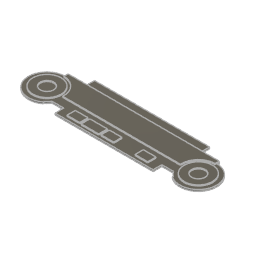
Face test plate (Autodesk Fusion 360 design; units mm, degrees)
Autodesk Fusion 360 part; units mm, degrees
sketch "Sketch1" plane through (0, 0, 0) normal (0, 0, 1) x (1, 0, 0)
  line L0 (110.9582, 1.828) -> (110.9582, -11.672)
  line L1 (-73.5418, 1.828) -> (-73.5418, -11.672)
  line L2 (-73.5418, -24.672) -> (110.9582, -24.672)
  line L3 (-73.5418, 15.328) -> (110.9582, 15.328)
  line L4 (110.9582, -24.672) -> (130.9582, -24.672)
  line L5 (130.9582, -24.672) -> (130.9582, -11.672)
  line L6 (130.9582, 15.328) -> (110.9582, 15.328)
  line L7 (-73.5418, 15.328) -> (-93.5418, 15.328)
  line L8 (-93.5418, -4.672) -> (-93.5418, -24.672)
  line L9 (-93.5418, -24.672) -> (-73.5418, -24.672)
  line L10 (130.9582, -4.672) -> (150.3831, -4.672)
  line L11 (130.9582, 15.328) -> (150.3831, 15.328)
  line L12 (-93.5418, -24.672) -> (-93.5418, -24)
  line L13 (-93.5418, -4.672) -> (-112.9667, -4.672)
  line L14 (-93.5418, 15.328) -> (-112.9667, 15.328)
  line L15 (130.9582, -4.672) -> (130.9582, -11.672)
  line L16 (-112.9667, 85.328) -> (-110, 85.328)
  line L17 (-110, 85.328) -> (150.3831, 85.328)
  line L18 (18.7082, 66.328) -> (150.3831, 66.328)
  line L19 (18.7082, 66.328) -> (16.2618, 66.328)
  line L20 (16.2618, 66.328) -> (-112.9667, 66.328)
  line L21 (157.4958, -4.672) -> (150.3831, -4.672)
  line L22 (191.7412, -4.672) -> (190, -4.672)
  line L23 (-112.9667, -4.672) -> (-120.0796, -4.672)
  circle A0 centre (191.7412, 17.8726) radius 32.5
  circle A1 centre (-154.3247, 17.873) radius 32.5
  line L24 (-112.9667, 66.328) -> (-154.3247, 66.328)
  line L25 (-154.3247, 66.328) -> (-154.3247, 60.373)
  line L26 (150.3831, 66.328) -> (191.7412, 66.328)
  line L27 (191.7412, 66.328) -> (191.7412, 60.3726)
  line L28 (150.3831, 66.328) -> (150.3831, 85.328)
  line L29 (150.3831, 15.328) -> (153.3253, 15.328)
  line L30 (191.7412, 60.3726) -> (191.7412, 56.3726)
  arc A2 (157.4958, -4.672) -> (166.8041, -14.672) centre (191.7412, 17.8726) ccw
  arc A3 (191.7412, 56.3726) -> (153.3253, 15.328) centre (191.7412, 17.8726) ccw
  line L31 (-112.9667, 66.328) -> (-112.9667, 85.328)
  line L32 (-154.3247, 60.373) -> (-154.3247, 56.373)
  line L33 (-112.9667, 15.328) -> (-115.9089, 15.328)
  arc A4 (-154.3247, 60.373) -> (-128.382, -15.7904) centre (-154.3247, 17.873) ccw
  arc A5 (-129.3883, -14.672) -> (-120.0796, -4.672) centre (-154.3247, 17.873) ccw
  arc A6 (-115.9089, 15.328) -> (-154.3247, 56.373) centre (-154.3247, 17.873) ccw
  line L34 (130.9582, -24.672) -> (130.9582, -14.672)
  line L35 (165.7979, -15.7904) -> (166.8041, -14.672)
  line L36 (-129.3883, -14.672) -> (-128.382, -15.7904)
  arc A7 (165.7979, -15.7904) -> (233.946, 12.8726) centre (191.7412, 17.8726) ccw
  arc A8 (233.946, 22.8726) -> (191.7412, 60.3726) centre (191.7412, 17.8726) ccw
  line L37 (110.9582, 1.828) -> (81.9582, 1.828)
  line L38 (81.9582, 1.828) -> (81.9582, -17.172)
  line L39 (81.9582, -17.172) -> (110.9582, -17.172)
  line L40 (110.9582, -17.172) -> (110.9582, -11.672)
  line L41 (-73.5418, 1.828) -> (-44.5418, 1.828)
  line L42 (-44.5418, 1.828) -> (-44.5418, -17.172)
  line L43 (-44.5418, -17.172) -> (-73.5418, -17.172)
  line L44 (-73.5418, -17.172) -> (-73.5418, -11.672)
  line L45 (33.2082, 1.828) -> (4.2082, 1.828)
  line L46 (33.2082, 1.828) -> (33.2082, -17.172)
  line L47 (33.2082, -17.172) -> (4.2082, -17.172)
  line L48 (4.2082, -17.172) -> (4.2082, 1.828)
  line L49 (-0.1668, 1.828) -> (-40.1668, 1.828)
  line L50 (-0.1668, 1.828) -> (-0.1668, -18.172)
  line L51 (-0.1668, -18.172) -> (-40.1668, -18.172)
  line L52 (-40.1668, -18.172) -> (-40.1668, 1.828)
  line L53 (233.946, 22.8726) -> (233.946, 12.8726)
  circle A9 centre (-154.3247, 17.873) radius 15.5
  circle A10 centre (191.7412, 17.8726) radius 15.5
  dimension "d9" = 13
  dimension "d10" = 13
  dimension "d12" = 13.5
  dimension "d13" = 13.5
  dimension "d14" = 20
  dimension "d15" = 20
  dimension "d16" = 20
  dimension "d17" = 20
  dimension "d50" = 70
  dimension "d51" = 70
  dimension "d57" = 65
  dimension "d58" = 77
  dimension "d59" = 65
  dimension "d60" = 77
  dimension "d61" = 82
  dimension "d63" = 82
  dimension "d64" = 85
  dimension "d65" = 10
  dimension "d68" = 29
  dimension "d69" = 19
  dimension "d70" = 29
  dimension "d71" = 19
  dimension "d73" = 29
  dimension "d74" = 19
  dimension "d76" = 40
  dimension "d77" = 20
  dimension "d78" = 40
  dimension "d79" = 31
  dimension "d80" = 31
  constraint vertical L0
  constraint vertical L1
  constraint perpendicular L2 L8
  constraint coincident L8 L12.end
  constraint perpendicular L9 L12
  constraint perpendicular L8 L13
  constraint perpendicular L8 L14
  constraint perpendicular L10 L15
  constraint perpendicular L16 L31
  constraint perpendicular L17 L28
  constraint perpendicular L18 L28
  constraint perpendicular L20 L31
  constraint coincident L21 L22.end
  constraint concentric A0 A3
  constraint concentric A1 A6
  constraint concentric A2 A3
  constraint concentric A1 A5
  constraint concentric A1 A4
  constraint horizontal L24
  constraint perpendicular L24 L25
  constraint perpendicular L25 L26
  constraint perpendicular L26 L27
  constraint vertical L30
  constraint vertical L32
  constraint perpendicular L4 L34
  constraint concentric A7 A8
  constraint perpendicular L0 L37
  constraint perpendicular L0 L39
  constraint perpendicular L1 L43
  constraint perpendicular L43 L44
  constraint perpendicular L46 L47
  constraint perpendicular L49 L50
  constraint perpendicular L50 L51
  constraint concentric A4 A9
  constraint concentric A2 A10
  measures "d9" distance of L0.end L2.end
  measures "d10" distance of L1.end L2.start
  measures "d12" distance of L0.start L3.end
  measures "d13" distance of L1.start L3.start
  measures "d14" distance of L0.end L5.end
  measures "d15" distance of L2.end L4.end
  measures "d16" distance of L3.start L7.end
  measures "d17" distance of L6.start L10.start
  measures "d50" distance of L11.end L17.end
  measures "d51" distance of L14.end L16.start
  measures "d57" diameter of A0
  measures "d58" diameter of A3
  measures "d59" diameter of A1
  measures "d60" diameter of A6
  measures "d61" diameter of A2
  measures "d63" diameter of A5
  measures "d64" diameter of A4
  measures "d65" distance of L4.end L34.end
  measures "d68" distance of L0.start L37.end
  measures "d69" distance of L37.end L38.end
  measures "d70" distance of L1.start L41.end
  measures "d71" distance of L41.end L42.end
  measures "d73" distance of L45.start L45.end
  measures "d74" distance of L45.start L46.end
  measures "d76" distance of L49.start L49.end
  measures "d77" distance of L49.start L50.end
  measures "d78" distance of L50.end L51.end
  measures "d79" diameter of A9
  measures "d80" diameter of A10
extrude "Extrude1" add sketch "Sketch1" along normal blind 4 contours L0 L37 L38 L39 L40 | L1 L41 L42 L43 L44 | L2 L3 L4 L5 L6 L7 L8 L9 L10 L11 L12 L13 L14 L15 L21 L23 L29 L30 A2 A3 L32 L33 A4 A5 A6 L34 L35 L36 A7 A8 L53 | L3 L6 L7 L11 L14 L18 L19 L20 L24 L25 L26 L27 L29 L30 A3 L32 L33 A6 | L16 L17 L18 L19 L20 L28 L31 | A0 | A1 | L45 L46 L47 L48 | L49 L50 L51 L52 | A9 | A10
sketch "Sketch2" plane through (0, 0, 4) normal (0, 0, 1) x (-1, 0, 0)
  line L0 (-150.3831, -66.328) -> (-150.3831, -85.328)
  line L1 (-150.3831, -85.328) -> (112.9667, -85.328)
  line L2 (112.9667, -85.328) -> (112.9667, -66.328)
  line L3 (112.9667, -66.328) -> (154.3247, -66.328)
  line L4 (154.3247, -66.328) -> (154.3247, -60.373)
  arc A0 (154.3247, -60.373) -> (128.382, 15.7904) centre (154.3247, -17.873) ccw
  line L5 (128.382, 15.7904) -> (129.3883, 14.672)
  arc A1 (129.3883, 14.672) -> (120.0796, 4.672) centre (154.3247, -17.873) ccw
  line L6 (120.0796, 4.672) -> (93.5418, 4.672)
  line L7 (93.5418, 4.672) -> (93.5418, 24.672)
  line L8 (93.5418, 24.672) -> (-130.9582, 24.672)
  line L9 (-130.9582, 24.672) -> (-130.9582, 4.672)
  line L10 (-130.9582, 4.672) -> (-157.4958, 4.672)
  arc A2 (-157.4958, 4.672) -> (-166.8041, 14.672) centre (-191.7412, -17.8726) ccw
  line L11 (-166.8041, 14.672) -> (-165.7979, 15.7904)
  arc A3 (-165.7979, 15.7904) -> (-233.946, -12.8726) centre (-191.7412, -17.8726) ccw
  line L12 (-233.946, -12.8726) -> (-233.946, -22.8726)
  arc A4 (-233.946, -22.8726) -> (-191.7412, -60.3726) centre (-191.7412, -17.8726) ccw
  line L13 (-191.7412, -60.3726) -> (-191.7412, -66.328)
  line L14 (-191.7412, -66.328) -> (-150.3831, -66.328)
  arc A5 (-191.6728, -56.4374) -> (-153.2569, -15.3929) centre (-191.6728, -17.9374) ccw
  line L15 (154.393, -66.3929) -> (154.393, -60.4379)
  line L16 (73.6102, -15.3929) -> (-110.8898, -15.3929)
  line L17 (113.035, -66.3929) -> (113.035, -85.3929)
  line L18 (40.2352, 18.1071) -> (40.2352, -1.8929)
  line L19 (110.0684, -85.3929) -> (-150.3147, -85.3929)
  line L20 (0.2352, 18.1071) -> (40.2352, 18.1071)
  line L21 (-33.1398, -1.8929) -> (-33.1398, 17.1071)
  line L22 (-16.1934, -66.3929) -> (113.035, -66.3929)
  arc A6 (154.393, -60.4379) -> (128.4504, 15.7255) centre (154.393, -17.9379) ccw
  line L23 (-18.6398, -66.3929) -> (-150.3147, -66.3929)
  line L24 (73.6102, 24.6071) -> (-110.8898, 24.6071)
  arc A7 (129.4567, 14.6071) -> (120.148, 4.6071) centre (154.393, -17.9379) ccw
  line L25 (113.035, -66.3929) -> (154.393, -66.3929)
  line L26 (73.6102, -15.3929) -> (93.6102, -15.3929)
  line L27 (113.035, -15.3929) -> (115.9772, -15.3929)
  line L28 (113.035, 4.6071) -> (120.148, 4.6071)
  line L29 (93.6102, 4.6071) -> (113.035, 4.6071)
  line L30 (93.6102, 24.6071) -> (93.6102, 23.9351)
  line L31 (44.6102, 17.1071) -> (73.6102, 17.1071)
  line L32 (93.6102, 4.6071) -> (93.6102, 24.6071)
  line L33 (0.2352, -1.8929) -> (0.2352, 18.1071)
  line L34 (73.6102, -1.8929) -> (44.6102, -1.8929)
  line L35 (93.6102, 24.6071) -> (73.6102, 24.6071)
  line L36 (73.6102, 17.1071) -> (73.6102, 11.6071)
  line L37 (-18.6398, -66.3929) -> (-16.1934, -66.3929)
  line L38 (129.4567, 14.6071) -> (128.4504, 15.7255)
  line L39 (73.6102, -1.8929) -> (73.6102, 11.6071)
  line L40 (154.393, -60.4379) -> (154.393, -56.4379)
  line L41 (-4.1398, 17.1071) -> (-4.1398, -1.8929)
  line L42 (44.6102, -1.8929) -> (44.6102, 17.1071)
  line L43 (113.035, -85.3929) -> (110.0684, -85.3929)
  line L44 (93.6102, -15.3929) -> (113.035, -15.3929)
  line L45 (-33.1398, 17.1071) -> (-4.1398, 17.1071)
  line L46 (-33.1398, -1.8929) -> (-4.1398, -1.8929)
  line L47 (0.2352, -1.8929) -> (40.2352, -1.8929)
  circle A8 centre (-191.6728, -17.9374) radius 15.5
  line L48 (-110.8898, -1.8929) -> (-81.8898, -1.8929)
  line L49 (-191.6728, -60.4374) -> (-191.6728, -56.4374)
  line L50 (-130.8898, 4.6071) -> (-150.3147, 4.6071)
  line L51 (-130.8898, -15.3929) -> (-110.8898, -15.3929)
  line L52 (-81.8898, -1.8929) -> (-81.8898, 17.1071)
  arc A9 (-233.8776, -22.9374) -> (-191.6728, -60.4374) centre (-191.6728, -17.9374) ccw
  circle A10 centre (-191.6728, -17.9374) radius 32.5
  line L53 (-130.8898, 24.6071) -> (-130.8898, 11.6071)
  arc A11 (-157.4274, 4.6071) -> (-166.7357, 14.6071) centre (-191.6728, -17.9374) ccw
  line L54 (-157.4274, 4.6071) -> (-150.3147, 4.6071)
  line L55 (-110.8898, 24.6071) -> (-130.8898, 24.6071)
  line L56 (-130.8898, -15.3929) -> (-150.3147, -15.3929)
  line L57 (-110.8898, 17.1071) -> (-110.8898, 11.6071)
  line L58 (-165.7295, 15.7255) -> (-166.7357, 14.6071)
  line L59 (-191.6728, -66.3929) -> (-191.6728, -60.4374)
  line L60 (-130.8898, 24.6071) -> (-130.8898, 14.6071)
  line L61 (-81.8898, 17.1071) -> (-110.8898, 17.1071)
  arc A12 (-165.7295, 15.7255) -> (-233.8776, -12.9374) centre (-191.6728, -17.9374) ccw
  line L62 (-150.3147, -15.3929) -> (-153.2569, -15.3929)
  line L63 (-233.8776, -22.9374) -> (-233.8776, -12.9374)
  line L64 (-110.8898, -1.8929) -> (-110.8898, 11.6071)
  line L65 (-150.3147, -66.3929) -> (-150.3147, -85.3929)
  line L66 (-130.8898, 4.6071) -> (-130.8898, 11.6071)
  line L67 (-150.3147, -66.3929) -> (-191.6728, -66.3929)
  circle A13 centre (154.393, -17.9379) radius 32.5
  circle A14 centre (154.393, -17.9379) radius 15.5
  arc A15 (115.9772, -15.3929) -> (154.393, -56.4379) centre (154.393, -17.9379) ccw
  point P0 (0.0684, -0.0649)
  dimension "d83" = 13
  dimension "d84" = 13
  dimension "d85" = 13.5
  dimension "d86" = 13.5
  dimension "d87" = 20
  dimension "d88" = 20
  dimension "d89" = 20
  dimension "d90" = 20
  dimension "d91" = 70
  dimension "d92" = 70
  dimension "d93" = 65
  dimension "d94" = 77
  dimension "d95" = 65
  dimension "d96" = 77
  dimension "d97" = 82
  dimension "d98" = 82
  dimension "d99" = 85
  dimension "d100" = 10
  dimension "d101" = 29
  dimension "d102" = 19
  dimension "d103" = 29
  dimension "d104" = 19
  dimension "d105" = 29
  dimension "d106" = 19
  dimension "d107" = 40
  dimension "d108" = 20
  dimension "d109" = 40
  dimension "d110" = 31
  dimension "d111" = 31
  constraint perpendicular L24 L32
  constraint coincident L30.end L32
  constraint perpendicular L30 L35
  constraint perpendicular L29 L32
  constraint perpendicular L32 L44
  constraint perpendicular L50 L66
  constraint perpendicular L17 L43
  constraint perpendicular L19 L65
  constraint perpendicular L23 L65
  constraint perpendicular L17 L22
  constraint concentric A5 A10
  constraint concentric A13 A15
  constraint concentric A5 A11
  constraint concentric A7 A13
  constraint concentric A6 A13
  constraint perpendicular L15 L25
  constraint perpendicular L15 L67
  constraint perpendicular L59 L67
  constraint perpendicular L55 L60
  constraint concentric A9 A12
  constraint perpendicular L48 L64
  constraint perpendicular L61 L64
  constraint perpendicular L31 L39
  constraint perpendicular L31 L36
  constraint perpendicular L21 L45
  constraint perpendicular L33 L47
  constraint perpendicular L20 L33
  constraint concentric A6 A14
  constraint concentric A8 A11
  measures "d83" distance of L24.end L57.end
  measures "d84" distance of L36.end L24.start
  measures "d85" distance of L48.start L16.end
  measures "d86" distance of L34.start L16.start
  measures "d87" distance of L57.end L53.end
  measures "d88" distance of L24.end L53.start
  measures "d89" distance of L16.start L26.end
  measures "d90" distance of L51.start L50.start
  measures "d91" distance of L19.end L56.end
  measures "d92" distance of L27.start L17.end
  measures "d93" diameter of A10
  measures "d94" diameter of A5
  measures "d95" diameter of A13
  measures "d96" diameter of A15
  measures "d97" diameter of A11
  measures "d98" diameter of A7
  measures "d99" diameter of A6
  measures "d100" distance of L53.start L60.end
  measures "d101" distance of L48.start L48.end
  measures "d102" distance of L48.end L52.end
  measures "d103" distance of L34.start L34.end
  measures "d104" distance of L34.end L31.start
  measures "d105" distance of L41.end L21.start
  measures "d106" distance of L21.end L21.start
  measures "d107" distance of L18.end L33.start
  measures "d108" distance of L20.start L33.start
  measures "d109" distance of L20.start L18.start
  measures "d110" diameter of A14
  measures "d111" diameter of A8
extrude "Extrude2" add sketch "Sketch2" along normal blind 2 contours L0 L2 L3 L4 A0 L14 A5 L16 L22 L23 L26 L27 L37 L40 L44 L49 L51 L56 L59 L62 L67 A15
sketch "Sketch3" plane through (0, 0, 4) normal (0, 0, 1) x (-1, 0, 0)
  line L0 (-191.6728, -66.328) -> (-191.6728, -56.4374)
  arc A0 (-191.6728, -56.4374) -> (-153.2569, -15.3929) centre (-191.6728, -17.9374) ccw
  line L1 (-153.2569, -15.3929) -> (115.9772, -15.3929)
  arc A1 (115.9772, -15.3929) -> (154.393, -56.4379) centre (154.393, -17.9379) ccw
  line L2 (154.393, -56.4379) -> (154.393, -60.373)
  arc A2 (154.393, -60.373) -> (128.382, 15.7904) centre (154.3247, -17.873) ccw
  line L3 (128.382, 15.7904) -> (129.3883, 14.672)
  arc A3 (129.3883, 14.672) -> (120.0796, 4.672) centre (154.3247, -17.873) ccw
  line L4 (120.0796, 4.672) -> (93.5418, 4.672)
  line L5 (93.5418, 4.672) -> (93.5418, 24.672)
  line L6 (93.5418, 24.672) -> (-130.9582, 24.672)
  line L7 (-130.9582, 24.672) -> (-130.9582, 4.672)
  line L8 (-130.9582, 4.672) -> (-157.4958, 4.672)
  arc A4 (-157.4958, 4.672) -> (-166.8041, 14.672) centre (-191.7412, -17.8726) ccw
  line L9 (-166.8041, 14.672) -> (-165.7979, 15.7904)
  arc A5 (-165.7979, 15.7904) -> (-233.946, -12.8726) centre (-191.7412, -17.8726) ccw
  line L10 (-233.946, -12.8726) -> (-233.946, -22.8726)
  arc A6 (-233.946, -22.8726) -> (-191.7412, -60.3726) centre (-191.7412, -17.8726) ccw
  line L11 (-191.7412, -60.3726) -> (-191.7412, -66.328)
  line L12 (-191.7412, -66.328) -> (-191.6728, -66.328)
  arc A7 (-191.7975, -56.4377) -> (-153.3817, -15.3932) centre (-191.7975, -17.9377) ccw
  line L13 (154.2683, -66.3932) -> (154.2683, -60.4382)
  line L14 (73.4855, -15.3932) -> (-111.0145, -15.3932)
  line L15 (112.9103, -66.3932) -> (112.9103, -85.3932)
  line L16 (40.1105, 18.1068) -> (40.1105, -1.8932)
  line L17 (109.9436, -85.3932) -> (-150.4395, -85.3932)
  line L18 (0.1105, 18.1068) -> (40.1105, 18.1068)
  line L19 (-33.2645, -1.8932) -> (-33.2645, 17.1068)
  line L20 (-16.3182, -66.3932) -> (112.9103, -66.3932)
  arc A8 (154.2683, -60.4382) -> (128.3256, 15.7252) centre (154.2683, -17.9382) ccw
  line L21 (-18.7645, -66.3932) -> (-150.4395, -66.3932)
  line L22 (73.4855, 24.6068) -> (-111.0145, 24.6068)
  arc A9 (129.3319, 14.6068) -> (120.0232, 4.6068) centre (154.2683, -17.9382) ccw
  line L23 (112.9103, -66.3932) -> (154.2683, -66.3932)
  line L24 (73.4855, -15.3932) -> (93.4855, -15.3932)
  line L25 (112.9103, -15.3932) -> (115.8525, -15.3932)
  line L26 (112.9103, 4.6068) -> (120.0232, 4.6068)
  line L27 (93.4855, 4.6068) -> (112.9103, 4.6068)
  line L28 (93.4855, 24.6068) -> (93.4855, 23.9348)
  line L29 (44.4855, 17.1068) -> (73.4855, 17.1068)
  line L30 (93.4855, 4.6068) -> (93.4855, 24.6068)
  line L31 (0.1105, -1.8932) -> (0.1105, 18.1068)
  line L32 (73.4855, -1.8932) -> (44.4855, -1.8932)
  line L33 (93.4855, 24.6068) -> (73.4855, 24.6068)
  line L34 (73.4855, 17.1068) -> (73.4855, 11.6068)
  line L35 (-18.7645, -66.3932) -> (-16.3182, -66.3932)
  line L36 (129.3319, 14.6068) -> (128.3256, 15.7252)
  line L37 (73.4855, -1.8932) -> (73.4855, 11.6068)
  line L38 (154.2683, -60.4382) -> (154.2683, -56.4382)
  line L39 (-4.2645, 17.1068) -> (-4.2645, -1.8932)
  line L40 (44.4855, -1.8932) -> (44.4855, 17.1068)
  line L41 (112.9103, -85.3932) -> (109.9436, -85.3932)
  line L42 (93.4855, -15.3932) -> (112.9103, -15.3932)
  line L43 (-33.2645, 17.1068) -> (-4.2645, 17.1068)
  line L44 (-33.2645, -1.8932) -> (-4.2645, -1.8932)
  line L45 (0.1105, -1.8932) -> (40.1105, -1.8932)
  circle A10 centre (-191.7975, -17.9377) radius 15.5
  line L46 (-111.0145, -1.8932) -> (-82.0145, -1.8932)
  line L47 (-191.7975, -60.4377) -> (-191.7975, -56.4377)
  line L48 (-131.0145, 4.6068) -> (-150.4395, 4.6068)
  line L49 (-131.0145, -15.3932) -> (-111.0145, -15.3932)
  line L50 (-82.0145, -1.8932) -> (-82.0145, 17.1068)
  arc A11 (-234.0024, -22.9377) -> (-191.7975, -60.4377) centre (-191.7975, -17.9377) ccw
  circle A12 centre (-191.7975, -17.9377) radius 32.5
  line L51 (-131.0145, 24.6068) -> (-131.0145, 11.6068)
  arc A13 (-157.5522, 4.6068) -> (-166.8605, 14.6068) centre (-191.7975, -17.9377) ccw
  line L52 (-157.5522, 4.6068) -> (-150.4395, 4.6068)
  line L53 (-111.0145, 24.6068) -> (-131.0145, 24.6068)
  line L54 (-131.0145, -15.3932) -> (-150.4395, -15.3932)
  line L55 (-111.0145, 17.1068) -> (-111.0145, 11.6068)
  line L56 (-165.8542, 15.7252) -> (-166.8605, 14.6068)
  line L57 (-191.7975, -66.3932) -> (-191.7975, -60.4377)
  line L58 (-131.0145, 24.6068) -> (-131.0145, 14.6068)
  line L59 (-82.0145, 17.1068) -> (-111.0145, 17.1068)
  arc A14 (-165.8542, 15.7252) -> (-234.0024, -12.9377) centre (-191.7975, -17.9377) ccw
  line L60 (-150.4395, -15.3932) -> (-153.3817, -15.3932)
  line L61 (-234.0024, -22.9377) -> (-234.0024, -12.9377)
  line L62 (-111.0145, -1.8932) -> (-111.0145, 11.6068)
  line L63 (-150.4395, -66.3932) -> (-150.4395, -85.3932)
  line L64 (-131.0145, 4.6068) -> (-131.0145, 11.6068)
  line L65 (-150.4395, -66.3932) -> (-191.7975, -66.3932)
  circle A15 centre (154.2683, -17.9382) radius 32.5
  circle A16 centre (154.2683, -17.9382) radius 15.5
  arc A17 (115.8525, -15.3932) -> (154.2683, -56.4382) centre (154.2683, -17.9382) ccw
  point P0 (-0.0564, -0.0652)
  dimension "d114" = 13
  dimension "d115" = 13
  dimension "d116" = 13.5
  dimension "d117" = 13.5
  dimension "d118" = 20
  dimension "d119" = 20
  dimension "d120" = 20
  dimension "d121" = 20
  dimension "d122" = 70
  dimension "d123" = 70
  dimension "d124" = 65
  dimension "d125" = 77
  dimension "d126" = 65
  dimension "d127" = 77
  dimension "d128" = 82
  dimension "d129" = 82
  dimension "d130" = 85
  dimension "d131" = 10
  dimension "d132" = 29
  dimension "d133" = 19
  dimension "d134" = 29
  dimension "d135" = 19
  dimension "d136" = 29
  dimension "d137" = 19
  dimension "d138" = 40
  dimension "d139" = 20
  dimension "d140" = 40
  dimension "d141" = 31
  dimension "d142" = 31
  constraint perpendicular L22 L30
  constraint coincident L28.end L30
  constraint perpendicular L28 L33
  constraint perpendicular L27 L30
  constraint perpendicular L30 L42
  constraint perpendicular L48 L64
  constraint perpendicular L15 L41
  constraint perpendicular L17 L63
  constraint perpendicular L21 L63
  constraint perpendicular L15 L20
  constraint concentric A7 A12
  constraint concentric A15 A17
  constraint concentric A7 A13
  constraint concentric A9 A15
  constraint concentric A8 A15
  constraint perpendicular L13 L23
  constraint perpendicular L13 L65
  constraint perpendicular L57 L65
  constraint perpendicular L53 L58
  constraint concentric A11 A14
  constraint perpendicular L46 L62
  constraint perpendicular L59 L62
  constraint perpendicular L29 L37
  constraint perpendicular L29 L34
  constraint perpendicular L19 L43
  constraint perpendicular L31 L45
  constraint perpendicular L18 L31
  constraint concentric A8 A16
  constraint concentric A10 A13
  measures "d114" distance of L22.end L55.end
  measures "d115" distance of L34.end L22.start
  measures "d116" distance of L46.start L14.end
  measures "d117" distance of L32.start L14.start
  measures "d118" distance of L55.end L51.end
  measures "d119" distance of L22.end L51.start
  measures "d120" distance of L14.start L24.end
  measures "d121" distance of L49.start L48.start
  measures "d122" distance of L17.end L54.end
  measures "d123" distance of L25.start L15.end
  measures "d124" diameter of A12
  measures "d125" diameter of A7
  measures "d126" diameter of A15
  measures "d127" diameter of A17
  measures "d128" diameter of A13
  measures "d129" diameter of A9
  measures "d130" diameter of A8
  measures "d131" distance of L51.start L58.end
  measures "d132" distance of L46.start L46.end
  measures "d133" distance of L46.end L50.end
  measures "d134" distance of L32.start L32.end
  measures "d135" distance of L32.end L29.start
  measures "d136" distance of L39.end L19.start
  measures "d137" distance of L19.end L19.start
  measures "d138" distance of L16.end L31.start
  measures "d139" distance of L18.start L31.start
  measures "d140" distance of L18.start L16.start
  measures "d141" diameter of A16
  measures "d142" diameter of A10
extrude "Extrude3" add sketch "Sketch3" along normal blind 2 contours L16 L18 L31 L45 | L19 L39 L43 L44 | L29 L32 L34 L37 L40 | L46 L50 L55 L59 L62 | A12 | A15
